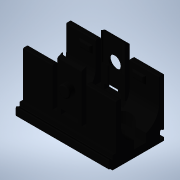
# Autodesk Inventor part: 653056 SDE5---(H)
Saved by Autodesk Inventor 2021 (Build 250183000, 183)
## iProperties
Created: 2026-04-21
Part Number: 653056 SDE5---(H)
Material: Generic
Catalog Web Link: www.3dfindit.com
Description: SDE5-(H)-Pressure sensors - Holder
Vendor: FESTO
Document SubType Name: Modeling
Designer: psAdmin
Manufacturer: FESTO
Mass: 6.71534 g
Surface Area: 62.7706 cm^2
Volume: 6.71534 cm^3
Density: 1 g/cm^3
Appearance: PSOLRGB-79-79-79
Category: PARTsolutions
Company: FESTO
Title: 653056 SDE5---(H)
Author: Cadenas PARTsolutions
Comments: Pressure sensors - Holder
PSOL_IDENT_0: {$CADENAS_DATA/23d-libs/festo/parts/s/sde5/parts/sde5_halter.prj},176 {VTYP=3D},{NB=653056 SDE5---(H
PSOL_IDENT_1: )},{LINA=653056 SDE5---(H)},{NN=SDE5-(H)},{DATE=22.08.2025 13:16:38},{GEOMDATE=31.07.2025 21:10:00},
PSOL_IDENT_2: {VERSION=},{LINEID=10},{WBVAR=},{WBNUMERIC=}  {NB=653056 SDE5---(H)},{LINA=653056 SDE5---(H)},{KT=DU
PSOL_IDENT_3: MMY},{TNR=653056},{TYP=SDE5}
NB: 653056 SDE5---(H)
NN: SDE5-(H)
NT: Pressure sensors - Holder
NBSYN: $TNR. $TYP.---(H)
LINA: 653056 SDE5---(H)
CATALOG: Festo
TNR: 653056
TYP: SDE5
SUPPLIER: FESTO
ARTICLENO: 653056 SDE5---(H)
BOMINFO: 653056 SDE5---(H)
CREATOR: CADENAS GmbH
Autodesk Inventor part; units mm, degrees
sketch "Skizze_1" plane through (0, 0, 0) normal (1, 0, 0) x (0, 1, 0)
  line L0 (4.1041, 13) -> (1.2959, 13)
  arc A0 (1.2959, 13) -> (1.036, 12.55) centre (1.2959, 12.7) ccw
  line L1 (1.036, 12.55) -> (1.5268, 11.7)
  arc A1 (1.3536, 11.4) -> (1.5268, 11.7) centre (1.3536, 11.6) ccw
  line L2 (1.3536, 11.4) -> (0, 11.4)
  line L3 (0, 11.4) -> (0, -10)
  line L4 (0, -10) -> (1.0804, -10)
  arc A2 (1.0804, -10) -> (1.3402, -9.55) centre (1.0804, -9.7) ccw
  line L5 (1.3402, -9.55) -> (0.9649, -8.9)
  arc A3 (1.3113, -8.3) -> (0.9649, -8.9) centre (1.3113, -8.7) ccw
  line L6 (1.3113, -8.3) -> (4.0887, -8.3)
  arc A4 (4.4351, -8.9) -> (4.0887, -8.3) centre (4.0887, -8.7) ccw
  line L7 (4.4351, -8.9) -> (4.0598, -9.55)
  arc A5 (4.0598, -9.55) -> (4.3196, -10) centre (4.3196, -9.7) ccw
  line L8 (4.3196, -10) -> (23.6, -10)
  arc A6 (23.6, -10) -> (24, -9.6) centre (23.6, -9.6) ccw
  line L9 (24, -9.6) -> (24, -8.3)
  arc A7 (24, -8.3) -> (23.6, -7.9) centre (23.6, -8.3) ccw
  line L10 (23.6, -7.9) -> (13.9, -7.9)
  arc A8 (13.9, 7.9) -> (13.9, -7.9) centre (13.9, 0) ccw
  line L11 (13.9, 7.9) -> (23.6, 7.9)
  arc A9 (23.6, 7.9) -> (24, 8.3) centre (23.6, 8.3) ccw
  line L12 (24, 8.3) -> (24, 9.6)
  arc A10 (24, 9.6) -> (23.6, 10) centre (23.6, 9.6) ccw
  line L13 (23.6, 10) -> (5.4, 10)
  line L14 (5.4, 10) -> (5.4, 11.4)
  line L15 (5.4, 11.4) -> (4.0464, 11.4)
  arc A11 (3.8732, 11.7) -> (4.0464, 11.4) centre (4.0464, 11.6) ccw
  line L16 (3.8732, 11.7) -> (4.364, 12.55)
  arc A12 (4.364, 12.55) -> (4.1041, 13) centre (4.1041, 12.7) ccw
  constraints: 34 end point, 26 point on circle, 13 centre point
extrude "Extrusion1" add sketch "Skizze_1" along normal mid plane 38.5
sketch "Skizze_2" plane through (0, 0, 0) normal (0, 0, 1) x (1, 0, 0)
  line L0 (-7, 33) -> (-7, 8)
  line L1 (-7, 8) -> (7, 8)
  line L2 (7, 8) -> (7, 33)
  line L3 (7, 33) -> (-7, 33)
  constraints: 8 end point
extrude "Extrusion2" cut sketch "Skizze_2" along normal mid plane 24
sketch "Skizze_3" plane through (0, 0, 0) normal (1, 0, 0) x (0, 1, 0)
  line L0 (28.5639, -8) -> (8, -8)
  line L1 (8, -8) -> (8, -10)
  line L2 (8, -10) -> (27.4019, -10)
  arc A0 (27.4019, -10) -> (27.7585, -9.7811) centre (27.4019, -9.6) ccw
  arc A1 (27.7585, -9.7811) -> (28.5639, -8) centre (8.5, 0) ccw
  constraints: 6 end point, 4 point on circle, 2 centre point
extrude "Extrusion3" add sketch "Skizze_3" along normal mid plane 10
sketch "Skizze_4" plane through (0, 0, 0) normal (1, 0, 0) x (0, 1, 0)
  line L0 (27.4019, 10) -> (8, 10)
  line L1 (8, 10) -> (8, 8)
  line L2 (8, 8) -> (28.5639, 8)
  arc A0 (28.5639, 8) -> (27.7585, 9.7811) centre (8.5, 0) ccw
  arc A1 (27.7585, 9.7811) -> (27.4019, 10) centre (27.4019, 9.6) ccw
  constraints: 6 end point, 4 point on circle, 2 centre point
extrude "Extrusion4" add sketch "Skizze_4" along normal mid plane 10
sketch "Skizze_5" plane through (0, 0, 0) normal (0, 0, 1) x (1, 0, 0)
  line L0 (-3.5, 10) -> (-3.5, 8)
  line L1 (-3.5, 8) -> (3.5, 8)
  line L2 (3.5, 8) -> (3.5, 10)
  line L3 (3.5, 10) -> (-3.5, 10)
  constraints: 8 end point
extrude "Extrusion5" cut sketch "Skizze_5" along normal mid plane 24
sketch "Skizze_6" plane through (0, 0, 0) normal (1, 0, 0) x (0, 1, 0)
  line L0 (19, 10) -> (19, 12.4)
  line L1 (19, 12.4) -> (20.9, 12.4)
  arc A0 (21.4, 11.9) -> (20.9, 12.4) centre (20.9, 11.9) ccw
  line L2 (21.4, 11.9) -> (21.4, 10)
  line L3 (21.4, 10) -> (19, 10)
  line L4 (19, 10) -> (19, 12.4)
  constraints: 10 end point, 2 point on circle, 1 centre point
revolve "Revolution1" add sketch "Skizze_6" angle 360 about axis through (0, 19, 10) along (0, 0, -1)
sketch "Sketch7" plane through (19.25, 4.3196, -10) normal (0, 0, -1) x (-1, 0, 0)
  point P0 (19.25, 14.6804)
hole "Hole1" at (0, 19, -10) direction (0, 0, 1) diameter 5 depth 2 countersink diameter 6 countersink angle 90
sketch "Skizze_8" plane through (8.25, 0, 0) normal (1, 0, 0) x (0, 0, -1)
  line L0 (7.2, 20.7994) -> (7.2, 19.2006)
  arc A0 (7.2, 19.2006) -> (7.45, 18.7675) centre (7.7, 19.2006) ccw
  line L1 (7.45, 18.7675) -> (7.75, 18.5943)
  arc A1 (8, 18.1613) -> (7.75, 18.5943) centre (7.5, 18.1613) ccw
  line L2 (8, 18.1613) -> (8, 21.8387)
  arc A2 (7.75, 21.4057) -> (8, 21.8387) centre (7.5, 21.8387) ccw
  line L3 (7.75, 21.4057) -> (7.45, 21.2325)
  arc A3 (7.45, 21.2325) -> (7.2, 20.7994) centre (7.7, 20.7994) ccw
  constraints: 8 end point, 8 point on circle, 4 centre point
extrude "Extrusion6" add sketch "Skizze_8" along normal blind 5.5
sketch "Skizze_9" plane through (8.25, 0, 0) normal (1, 0, 0) x (0, 0, -1)
  arc A0 (-7.75, 18.5943) -> (-8, 18.1613) centre (-7.5, 18.1613) ccw
  line L0 (-7.75, 18.5943) -> (-7.45, 18.7675)
  arc A1 (-7.45, 18.7675) -> (-7.2, 19.2006) centre (-7.7, 19.2006) ccw
  line L1 (-7.2, 19.2006) -> (-7.2, 20.7994)
  arc A2 (-7.2, 20.7994) -> (-7.45, 21.2325) centre (-7.7, 20.7994) ccw
  line L2 (-7.45, 21.2325) -> (-7.75, 21.4057)
  arc A3 (-8, 21.8387) -> (-7.75, 21.4057) centre (-7.5, 21.8387) ccw
  line L3 (-8, 21.8387) -> (-8, 18.1613)
  constraints: 8 end point, 8 point on circle, 4 centre point
extrude "Extrusion7" add sketch "Skizze_9" along normal blind 5.5
sketch "Skizze_10" plane through (-8.25, 0, 0) normal (1, 0, 0) x (0, 0, -1)
  line L0 (7.2, 20.7994) -> (7.2, 19.2006)
  arc A0 (7.2, 19.2006) -> (7.45, 18.7675) centre (7.7, 19.2006) ccw
  line L1 (7.45, 18.7675) -> (7.75, 18.5943)
  arc A1 (8, 18.1613) -> (7.75, 18.5943) centre (7.5, 18.1613) ccw
  line L2 (8, 18.1613) -> (8, 21.8387)
  arc A2 (7.75, 21.4057) -> (8, 21.8387) centre (7.5, 21.8387) ccw
  line L3 (7.75, 21.4057) -> (7.45, 21.2325)
  arc A3 (7.45, 21.2325) -> (7.2, 20.7994) centre (7.7, 20.7994) ccw
  constraints: 8 end point, 8 point on circle, 4 centre point
extrude "Extrusion8" add sketch "Skizze_10" against normal blind 5.5
sketch "Skizze_11" plane through (-8.25, 0, 0) normal (1, 0, 0) x (0, 0, -1)
  arc A0 (-7.75, 18.5943) -> (-8, 18.1613) centre (-7.5, 18.1613) ccw
  line L0 (-7.75, 18.5943) -> (-7.45, 18.7675)
  arc A1 (-7.45, 18.7675) -> (-7.2, 19.2006) centre (-7.7, 19.2006) ccw
  line L1 (-7.2, 19.2006) -> (-7.2, 20.7994)
  arc A2 (-7.2, 20.7994) -> (-7.45, 21.2325) centre (-7.7, 20.7994) ccw
  line L2 (-7.45, 21.2325) -> (-7.75, 21.4057)
  arc A3 (-8, 21.8387) -> (-7.75, 21.4057) centre (-7.5, 21.8387) ccw
  line L3 (-8, 21.8387) -> (-8, 18.1613)
  constraints: 8 end point, 8 point on circle, 4 centre point
extrude "Extrusion9" add sketch "Skizze_11" against normal blind 5.5
sketch "Skizze_12" plane through (0, 3, 0) normal (0, 1, 0) x (1, 0, 0)
  arc A0 (9.5, 5) -> (9.5, -5) centre (9.5, 0) ccw
  line L0 (9.5, -5) -> (10.5, -5)
  arc A1 (10.5, -5) -> (14.8301, -2.5) centre (10.5, 0) ccw
  line L1 (14.8301, -2.5) -> (19.25, -2.5)
  line L2 (19.25, -2.5) -> (19.25, 2.5)
  line L3 (19.25, 2.5) -> (14.8301, 2.5)
  arc A2 (14.8301, 2.5) -> (10.5, 5) centre (10.5, 0) ccw
  line L4 (10.5, 5) -> (9.5, 5)
  constraints: 10 end point, 6 point on circle, 3 centre point
extrude "Extrusion10" cut sketch "Skizze_12" along normal blind 7
sketch "Skizze_13" plane through (0, 3, 0) normal (0, 1, 0) x (1, 0, 0)
  line L0 (-19.25, -2.5) -> (-14.5826, -2.5)
  arc A0 (-14.5826, -2.5) -> (-5, -0.5) centre (-10, -0.5) ccw
  line L1 (-5, -0.5) -> (-5, 0.5)
  arc A1 (-5, 0.5) -> (-14.5826, 2.5) centre (-10, 0.5) ccw
  line L2 (-14.5826, 2.5) -> (-19.25, 2.5)
  line L3 (-19.25, 2.5) -> (-19.25, -2.5)
  constraints: 8 end point, 4 point on circle, 2 centre point
extrude "Extrusion11" cut sketch "Skizze_13" along normal blind 7
sketch "Skizze_14" plane through (0, 20, 0) normal (0, 1, 0) x (1, 0, 0)
  line L0 (8.25, 7.9) -> (8.25, 4.9)
  line L1 (8.25, 4.9) -> (13.75, 4.9)
  line L2 (13.75, 4.9) -> (13.75, 7.9)
  arc A0 (12.5262, 7.1) -> (13.75, 7.9) centre (12.2381, 8.8768) ccw
  line L3 (12.5262, 7.1) -> (9.4738, 7.1)
  arc A1 (8.25, 7.9) -> (9.4738, 7.1) centre (9.7619, 8.8768) ccw
  constraints: 8 end point, 4 point on circle, 2 centre point
extrude "Extrusion12" cut sketch "Skizze_14" along normal mid plane 5
sketch "Skizze_15" plane through (0, 20, 0) normal (0, 1, 0) x (1, 0, 0)
  line L0 (-13.75, 7.9) -> (-13.75, 4.9)
  line L1 (-13.75, 4.9) -> (-8.25, 4.9)
  line L2 (-8.25, 4.9) -> (-8.25, 7.9)
  arc A0 (-9.4738, 7.1) -> (-8.25, 7.9) centre (-9.7619, 8.8768) ccw
  line L3 (-9.4738, 7.1) -> (-12.5262, 7.1)
  arc A1 (-13.75, 7.9) -> (-12.5262, 7.1) centre (-12.2381, 8.8768) ccw
  constraints: 8 end point, 4 point on circle, 2 centre point
extrude "Extrusion13" cut sketch "Skizze_15" along normal mid plane 5
sketch "Skizze_16" plane through (0, 20, 0) normal (0, 1, 0) x (1, 0, 0)
  arc A0 (9.4738, -7.1) -> (8.25, -7.9) centre (9.7619, -8.8768) ccw
  line L0 (9.4738, -7.1) -> (12.5262, -7.1)
  arc A1 (13.75, -7.9) -> (12.5262, -7.1) centre (12.2381, -8.8768) ccw
  line L1 (13.75, -7.9) -> (13.75, -4.9)
  line L2 (13.75, -4.9) -> (8.25, -4.9)
  line L3 (8.25, -4.9) -> (8.25, -7.9)
  constraints: 8 end point, 4 point on circle, 2 centre point
extrude "Extrusion14" cut sketch "Skizze_16" along normal mid plane 5
sketch "Skizze_17" plane through (0, 20, 0) normal (0, 1, 0) x (1, 0, 0)
  arc A0 (-12.5262, -7.1) -> (-13.75, -7.9) centre (-12.2381, -8.8768) ccw
  line L0 (-12.5262, -7.1) -> (-9.4738, -7.1)
  arc A1 (-8.25, -7.9) -> (-9.4738, -7.1) centre (-9.7619, -8.8768) ccw
  line L1 (-8.25, -7.9) -> (-8.25, -4.9)
  line L2 (-8.25, -4.9) -> (-13.75, -4.9)
  line L3 (-13.75, -4.9) -> (-13.75, -7.9)
  constraints: 8 end point, 4 point on circle, 2 centre point
extrude "Extrusion15" cut sketch "Skizze_17" along normal mid plane 5
sketch "Skizze_18" plane through (0, 0, 0) normal (0, 1, 0) x (-1, 0, 0)
  line L0 (18.25, -6.8) -> (18.25, 8.5)
  line L1 (18.25, 8.5) -> (-18.25, 8.5)
  line L2 (-18.25, 8.5) -> (-18.25, -6.8)
  line L3 (-18.25, -6.8) -> (18.25, -6.8)
  constraints: 8 end point
extrude "Extrusion16" cut sketch "Skizze_18" along normal blind 1.5
sketch "Skizze_19" plane through (0, 17.1, 0) normal (0, 1, 0) x (1, 0, 0)
  line L0 (-4.675, 8.1782) -> (-4.675, -8.1782)
  arc A0 (-4.675, -8.1782) -> (-4.4189, -8.475) centre (-4.375, -8.1782) ccw
  arc A1 (-4.4189, -8.475) -> (4.4189, -8.475) centre (0, 21.4) ccw
  arc A2 (4.4189, -8.475) -> (4.675, -8.1782) centre (4.375, -8.1782) ccw
  line L1 (4.675, -8.1782) -> (4.675, 8.1782)
  arc A3 (4.675, 8.1782) -> (4.4189, 8.475) centre (4.375, 8.1782) ccw
  arc A4 (4.4189, 8.475) -> (-4.4189, 8.475) centre (0, -21.4) ccw
  arc A5 (-4.4189, 8.475) -> (-4.675, 8.1782) centre (-4.375, 8.1782) ccw
  constraints: 12 point on circle, 6 centre point, 4 end point
extrude "Extrusion17" cut sketch "Skizze_19" along normal blind 15
sketch "Skizze_20" plane through (0, 17.1, 0) normal (0, 1, 0) x (1, 0, 0)
  line L0 (-2.125, -8.7) -> (2.125, -8.7)
  line L1 (2.125, -8.7) -> (2.125, 8.7)
  line L2 (2.125, 8.7) -> (-2.125, 8.7)
  line L3 (-2.125, 8.7) -> (-2.125, -8.7)
  constraints: 8 end point
extrude "Extrusion18" cut sketch "Skizze_20" against normal blind 8
sketch "Skizze_21" plane through (0, 5, 0) normal (0, 1, 0) x (1, 0, 0)
  arc A0 (-2.125, -5.25) -> (-1.125, -6.25) centre (-1.125, -5.25) ccw
  line L0 (-1.125, -6.25) -> (1.125, -6.25)
  arc A1 (1.125, -6.25) -> (2.125, -5.25) centre (1.125, -5.25) ccw
  line L1 (2.125, -5.25) -> (2.125, 5.25)
  arc A2 (2.125, 5.25) -> (1.125, 6.25) centre (1.125, 5.25) ccw
  line L2 (1.125, 6.25) -> (-1.125, 6.25)
  arc A3 (-1.125, 6.25) -> (-2.125, 5.25) centre (-1.125, 5.25) ccw
  line L3 (-2.125, 5.25) -> (-2.125, -5.25)
  constraints: 8 end point, 8 point on circle, 4 centre point
extrude "Extrusion19" cut sketch "Skizze_21" along normal blind 7
sketch "Skizze_22" plane through (0, 0, 0) normal (0, 1, 0) x (-1, 0, 0)
  arc A0 (-9.5, -2.25) -> (-9.5, 2.25) centre (-9.5, 0) ccw
  line L0 (-9.5, 2.25) -> (-10.5, 2.25)
  arc A1 (-10.5, 2.25) -> (-10.5, -2.25) centre (-10.5, 0) ccw
  line L1 (-10.5, -2.25) -> (-9.5, -2.25)
  constraints: 4 end point, 4 point on circle, 2 centre point
extrude "Extrusion20" cut sketch "Skizze_22" along normal blind 7
sketch "Skizze_23" plane through (0, 0, 0) normal (0, 1, 0) x (-1, 0, 0)
  arc A0 (-9.5, -3.75) -> (-9.5, 3.75) centre (-9.5, 0) ccw
  line L0 (-9.5, 3.75) -> (-10.5, 3.75)
  arc A1 (-10.5, 3.75) -> (-10.5, -3.75) centre (-10.5, 0) ccw
  line L1 (-10.5, -3.75) -> (-9.5, -3.75)
  arc A2 (-9.5, -2.25) -> (-9.5, 2.25) centre (-9.5, 0) ccw
  line L2 (-9.5, 2.25) -> (-10.5, 2.25)
  arc A3 (-10.5, 2.25) -> (-10.5, -2.25) centre (-10.5, 0) ccw
  line L3 (-10.5, -2.25) -> (-9.5, -2.25)
  constraints: 8 end point, 8 point on circle, 4 centre point
extrude "Extrusion21" add sketch "Skizze_23" along normal blind 1.5
sketch "Skizze_24" plane through (0, 0, 0) normal (0, 1, 0) x (-1, 0, 0)
  line L0 (12.25, -0.5) -> (12.25, 0.5)
  arc A0 (12.25, 0.5) -> (7.75, 0.5) centre (10, 0.5) ccw
  line L1 (7.75, 0.5) -> (7.75, -0.5)
  arc A1 (7.75, -0.5) -> (12.25, -0.5) centre (10, -0.5) ccw
  constraints: 4 end point, 4 point on circle, 2 centre point
extrude "Extrusion22" cut sketch "Skizze_24" along normal blind 4
sketch "Skizze_25" plane through (0, 0, 0) normal (0, 1, 0) x (-1, 0, 0)
  arc A0 (13.75, 0.5) -> (6.25, 0.5) centre (10, 0.5) ccw
  line L0 (6.25, 0.5) -> (6.25, -0.5)
  arc A1 (6.25, -0.5) -> (13.75, -0.5) centre (10, -0.5) ccw
  line L1 (13.75, -0.5) -> (13.75, 0.5)
  arc A2 (12.25, 0.5) -> (7.75, 0.5) centre (10, 0.5) ccw
  line L2 (7.75, 0.5) -> (7.75, -0.5)
  arc A3 (7.75, -0.5) -> (12.25, -0.5) centre (10, -0.5) ccw
  line L3 (12.25, -0.5) -> (12.25, 0.5)
  constraints: 8 end point, 8 point on circle, 4 centre point
extrude "Extrusion23" add sketch "Skizze_25" along normal blind 1.5
ref_plane "ANBAU_XY" through (0, 14, 0) normal (1, 0, 0) x (0, 0, -1)
ref_plane "ANBAU_YZ" through (0, 14, 0) normal (0, 0, -1) x (0, 1, 0)
ref_plane "ANBAU_ZX" through (0, 14, 0) normal (0, 1, 0) x (1, 0, 0)
ref_plane "SPAF_XY" through (0, 13.9, 0) normal (1, 0, 0) x (0, 0, -1)
ref_plane "SPAF_YZ" through (0, 13.9, 0) normal (0, 0, -1) x (0, 1, 0)
ref_plane "SPAF_ZX" through (0, 13.9, 0) normal (0, 1, 0) x (1, 0, 0)
body "Solid1"
